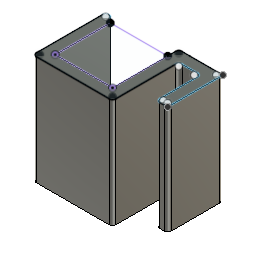
Nintendo switch wesa rail mount (Autodesk Fusion 360 design; units mm, degrees)
part number: 2025-12-19-15-03-05-764
Autodesk Fusion 360 part; units mm, degrees
note: some values were not read from the file. Set by a fixed rule: which sketch regions a step uses.
sketch "Sketch1" plane through (0, 0, 0) normal (0, 0, 1) x (1, 0, 0)
  line L0 (0, 0) -> (52, 0)
  line L1 (52, 0) -> (52, 50)
  line L2 (52, 50) -> (0, 50)
  line L3 (0, 50) -> (0, 0)
  dimension "d1" = 52
  dimension "d2" = 50
  constraint horizontal L0
  constraint vertical L1
  constraint horizontal L2
  constraint vertical L3
  constraint coincident L0.start L3.end
  measures "d1" distance of L0.start L0.end
  measures "d2" distance of L0.end L1.end
extrude "Extrude1" add sketch "Sketch1" along normal blind 99 makes body 1
sketch "Sketch2" plane through (0, 0, 99) normal (0, 0, 1) x (-1, 0, 0)
  line L0 (0, -50) -> (0, 0)
  line L1 (0, 0) -> (-52, 0)
  line L2 (-52, 0) -> (-52, -50)
  line L3 (-52, -50) -> (0, -50)
  line L4 (10, -52.7574) -> (10, 7)
  line L5 (7, 10) -> (-59, 10)
  line L6 (-62, 7) -> (-62, -47)
  line L7 (-62, -60) -> (-55, -60)
  line L8 (0, -50) -> (4.8787, -54.8787)
  line L9 (-62, -60) -> (-89, -60)
  line L10 (-92, -57) -> (-92, -13)
  line L11 (-89, -10) -> (-85, -10)
  line L12 (-82, -13) -> (-82, -47)
  line L13 (-79, -50) -> (-65, -50)
  line L14 (-52, -50) -> (-52, -57)
  arc A0 (-55, -60) -> (-52, -57) centre (-55, -57) ccw
  arc A1 (-65, -50) -> (-62, -47) centre (-65, -47) ccw
  arc A2 (-92, -57) -> (-89, -60) centre (-89, -57) ccw
  arc A3 (-82, -47) -> (-79, -50) centre (-79, -47) ccw
  arc A4 (-82, -13) -> (-85, -10) centre (-85, -13) ccw
  arc A5 (-89, -10) -> (-92, -13) centre (-89, -13) ccw
  arc A6 (-59, 10) -> (-62, 7) centre (-59, 7) ccw
  arc A7 (10, 7) -> (7, 10) centre (7, 7) ccw
  arc A8 (4.8787, -54.8787) -> (10, -52.7574) centre (7, -52.7574) ccw
  point P0 (-92, -60)
  point P1 (-92, -10)
  dimension "d8" = 30
  dimension "d9" = 50
  dimension "d10" = 3
  constraint coincident L0.start L3.end
  constraint perpendicular L6 L9
  constraint perpendicular L9 L10
  constraint perpendicular L10 L11
  constraint perpendicular L3 L12
  constraint perpendicular L6 L13
  constraint coincident L2.end L3.start
  constraint perpendicular L7 L14
  constraint tangent L14 A0
  constraint tangent L7 A0
  constraint tangent L13 A1
  constraint tangent L6 A1
  constraint equal A0 A1
  constraint coincident P0 L9
  constraint coincident P0 L10
  constraint tangent L9 A2
  constraint tangent L10 A2
  constraint equal A0 A2
  constraint tangent L12 A3
  constraint tangent L13 A3
  constraint equal A0 A3
  constraint tangent L11 A4
  constraint tangent L12 A4
  constraint equal A0 A4
  constraint coincident P1 L10
  constraint coincident P1 L11
  constraint tangent L10 A5
  constraint tangent L11 A5
  constraint equal A0 A5
  constraint tangent L5 A6
  constraint tangent L6 A6
  constraint equal A0 A6
  constraint tangent L4 A7
  constraint tangent L5 A7
  constraint equal A0 A7
  constraint tangent L4 A8
  constraint tangent L8 A8
  constraint equal A0 A8
  measures "d8" distance of L7.start P0
  measures "d9" distance of P0 P1
  measures "d10" radius of A0
extrude "Extrude2" add sketch "Sketch2" against normal blind 99 separate body contours L0 L1 L2 L4 L5 L6 L7 L8 L9 L10 L11 L12 L13 L14 A0 A1 A2 A3 A4 A5 A6 A7 A8 makes body 2
hidden bodies 1
named bodies: "HolderBody"
